Electrode Case Cap (Autodesk Fusion 360 design; units mm, degrees)
Autodesk Fusion 360 part; units mm, degrees
sketch "Sketch1" plane through (0, 0, 0) normal (0, 0, 1) x (1, 0, 0)
  circle A0 centre (0, 0) radius 9.25
  dimension "d1" = 18.5
  constraint coincident A0.centre origin
  measures "d1" diameter of A0
extrude "Extrude1" add sketch "Sketch1" along normal blind 1
sketch "Sketch2" plane through (0, 0, 1) normal (0, 0, 1) x (-1, 0, 0)
  circle A0 centre (0, 0) radius 9.25
  circle A1 centre (0, 0) radius 7
  dimension "d4" = 14
  constraint coincident A0.centre A1.centre
  measures "d4" diameter of A1
extrude "Extrude2" add sketch "Sketch2" along normal blind 2 contours A1
thread "Thread1" "ISO Metric profile 17.0 M17x1.5 M17x1.5 6g" major diameter 16.85 minor diameter 15.1369 pitch 1.5 angle 60 modelled right hand crest width 0.2152 on face at (-6.9652, 0.697, 2.3333) crest through (-8.425, 0, 0.625)
fillet "Fillet1" radius 0.5 1 edges at (-8.624, -3.3449, 0)
sketch "Sketch3" plane through (0, 0, 3) normal (0, 0, 1) x (-1, 0, 0)
  spline S0 degree 3 poles (3.1399, 6.8864) (2.2591, 7.3476) (1.2959, 7.6306) (-0.7053, 7.8172) (-1.7248, 7.7112) (-3.6872, 7.1119) (-4.6088, 6.6168) (-6.2291, 5.2909) (-6.9072, 4.4667) (-7.7504, 2.9069) (-8.0069, 2.2356) (-8.3435, 0.8351) (-8.4199, 0.1112) (-8.4026, -0.6135) knots 0 0 0 0 0.298289 0.298289 0.602722 0.602722 0.913299 0.913299 1.230015 1.230015 1.44431 1.44431 1.661348 1.661348 1.661348 1.661348
  arc A0 (-8.4026, -0.6135) -> (-4.7326, -6.9701) centre (0, 0) ccw
  spline S1 degree 3 poles (-4.7326, -6.9701) (-3.8057, -7.5352) (-2.7782, -7.9155) (-0.6552, -8.2538) (0.4186, -8.2163) (2.4703, -7.7328) (3.4302, -7.2991) (5.1106, -6.0972) (5.8195, -5.347) (6.7186, -3.9145) (6.9995, -3.3044) (7.3932, -2.0356) (7.5066, -1.383) (7.5337, -0.7239) knots 0 0 0 0 0.32568 0.32568 0.645209 0.645209 0.958585 0.958585 1.265805 1.265805 1.46682 1.46682 1.665086 1.665086 1.665086 1.665086
  arc A1 (7.5337, -0.7239) -> (3.1399, 6.8864) centre (0, 0) ccw
  circle A2 centre (0, 0) radius 6.5
  dimension "d11" = 13
  constraint coincident A0.centre A1.centre
  measures "d11" diameter of A2
extrude "Extrude3" cut sketch "Sketch3" against normal blind 1 contours A2
